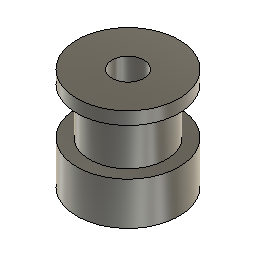
79d08786-4967-4a0b-b894-2fc37a93b006 (Autodesk Fusion 360 design; units mm, degrees)
Autodesk Fusion 360 part; units mm, degrees
sketch "Sketch1" plane through (0, 0, 0) normal (0, 0, 1) x (1, 0, 0)
  circle A0 centre (0, 0) radius 8
  circle A1 centre (0, 0) radius 2.5
  circle A2 centre (0, 0) radius 6
  dimension "d1" = 16
  dimension "d2" = 5
  dimension "d3" = 12
  constraint coincident A0.centre A1.centre
  constraint concentric A0 A1
  constraint concentric A1 A2
  measures "d1" diameter of A0
  measures "d2" diameter of A1
  measures "d3" diameter of A2
extrude "Extrude1" add sketch "Sketch1" along normal blind 6.7 contours A0 | A2
extrude "Extrude2" add sketch "Sketch1" along normal blind 16 contours A2
extrude "Extrude3" add sketch "Sketch1" against normal blind 2 from surface at 16 contours A0
equation "d4 = 16 mm - 7.3 mm - 2 mm"
